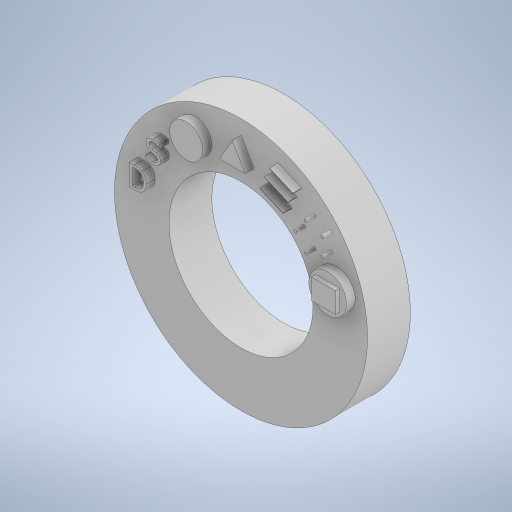
# Autodesk Inventor part: lab5CADfiguras
Saved by Autodesk Inventor 2023 (Build 270158000, 158)
## iProperties
Created: 2022-10-28
Part Number: lab5CADfiguras
Material: Generic
Document SubType Name: Modeling
Designer: jhair
Density: 1 g/cm^3
Appearance: Default
Author: jhair
Autodesk Inventor part; units mm, degrees
ref_plane "YZ Plane" through (0, 0, 0) normal (1, 0, 0) x (0, 1, 0)
ref_plane "XZ Plane" through (0, 0, 0) normal (0, 1, 0) x (-1, 0, 0)
ref_plane "XY Plane" through (0, 0, 0) normal (0, 0, 1) x (1, 0, 0)
sketch "Sketch1" plane through (0, 0, 0) normal (0, 0, 1) x (1, 0, 0)
  circle A0 centre (0, 0) radius 295
  circle A1 centre (0, 0) radius 168
  dimension "d0" = 590
  dimension "d1" = 336
  constraints: 2 centre point, 2 coincident
  measures "d0" diameter of A0
  measures "d1" diameter of A1
extrude "Extrusion1" add sketch "Sketch1" along normal blind 100
sketch "Sketch2" plane through (0, 0, 100) normal (0, 0, 1) x (1, 0, 0)
  line L0 (-204.3933, 171.1712) -> (-160.5291, 171.1712) construction
  line L1 (-160.5291, 171.1712) -> (-160.5291, 111.0696) construction
  line L2 (-160.5291, 111.0696) -> (-204.3933, 111.0696) construction
  line L3 (-204.3933, 111.0696) -> (-204.3933, 171.1712) construction
  line L4 (-245.1262, 97.2034) -> (-201.262, 97.2034) construction
  line L5 (-201.262, 97.2034) -> (-201.262, 37.1018) construction
  line L6 (-201.262, 37.1018) -> (-245.1262, 37.1018) construction
  line L7 (-245.1262, 37.1018) -> (-245.1262, 97.2034) construction
  spline S0 degree 2 poles (-185.39, 119.3884) (-190.8195, 119.3884) (-198.437, 121.6574) (-201.8001, 123.2782) knots 0 0 0 1 2 2 2
  line L8 (-201.8001, 123.2782) -> (-201.8001, 131.625)
  line L9 (-201.8001, 131.625) -> (-201.3139, 131.625)
  spline S1 degree 2 poles (-201.3139, 131.625) (-198.0319, 128.5456) (-189.7255, 125.142) (-185.8763, 125.142) knots 0 0 0 1 2 2 2
  spline S2 degree 2 poles (-185.8763, 125.142) (-180.3657, 125.142) (-174.7336, 129.7206) (-174.7336, 133.4889) knots 0 0 0 1 2 2 2
  spline S3 degree 2 poles (-174.7336, 133.4889) (-174.7336, 136.4873) (-177.6915, 140.215) (-180.8925, 141.1469) knots 0 0 0 1 2 2 2
  spline S4 degree 2 poles (-180.8925, 141.1469) (-183.202, 141.7952) (-187.0513, 142.6866) (-189.9281, 143.4159) knots 0 0 0 1 2 2 2
  spline S5 degree 2 poles (-189.9281, 143.4159) (-192.5213, 144.1048) (-196.6137, 146.1712) (-198.1939, 147.8325) knots 0 0 0 1 2 2 2
  spline S6 degree 2 poles (-198.1939, 147.8325) (-199.7336, 149.4937) (-201.4354, 153.9508) (-201.4354, 156.8681) knots 0 0 0 1 2 2 2
  spline S7 degree 2 poles (-201.4354, 156.8681) (-201.4354, 162.9459) (-191.9541, 171.1712) (-184.6202, 171.1712) knots 0 0 0 1 2 2 2
  spline S8 degree 2 poles (-184.6202, 171.1712) (-180.4062, 171.1712) (-172.9508, 169.51) (-169.7498, 167.9297) knots 0 0 0 1 2 2 2
  line L10 (-169.7498, 167.9297) -> (-169.7498, 159.9881)
  line L11 (-169.7498, 159.9881) -> (-170.2361, 159.9881)
  spline S9 degree 2 poles (-170.2361, 159.9881) (-172.6267, 162.1761) (-180.0821, 165.4176) (-184.1745, 165.4176) knots 0 0 0 1 2 2 2
  spline S10 degree 2 poles (-184.1745, 165.4176) (-188.7936, 165.4176) (-194.5067, 161.0821) (-194.5067, 157.557) knots 0 0 0 1 2 2 2
  spline S11 degree 2 poles (-194.5067, 157.557) (-194.5067, 154.3965) (-191.1437, 150.6283) (-187.9832, 149.7774) knots 0 0 0 1 2 2 2
  spline S12 degree 2 poles (-187.9832, 149.7774) (-185.8763, 149.2101) (-179.758, 147.7514) (-177.732, 147.1437) knots 0 0 0 1 2 2 2
  spline S13 degree 2 poles (-177.732, 147.1437) (-172.5862, 145.5634) (-167.805, 139.202) (-167.805, 134.5424) knots 0 0 0 1 2 2 2
  spline S14 degree 2 poles (-167.805, 134.5424) (-167.805, 131.5845) (-170.1956, 125.9119) (-172.343, 123.9265) knots 0 0 0 1 2 2 2
  spline S15 degree 2 poles (-172.343, 123.9265) (-174.7336, 121.7385) (-180.8114, 119.3884) (-185.39, 119.3884) knots 0 0 0 1 2 2 2
  spline S16 degree 2 poles (-200.6367, 72.1629) (-200.6367, 65.3152) (-206.1877, 54.2942) (-210.8474, 51.2147) knots 0 0 0 1 2 2 2
  spline S17 degree 2 poles (-210.8474, 51.2147) (-214.6561, 48.8241) (-222.4762, 47.2034) (-228.554, 47.2034) knots 0 0 0 1 2 2 2
  line L12 (-228.554, 47.2034) -> (-240.0613, 47.2034)
  line L13 (-240.0613, 47.2034) -> (-240.0613, 97.2034)
  line L14 (-240.0613, 97.2034) -> (-228.6756, 97.2034)
  spline S18 degree 2 poles (-228.6756, 97.2034) (-221.6253, 97.2034) (-213.6027, 95.0964) (-210.7663, 93.2326) knots 0 0 0 1 2 2 2
  spline S19 degree 2 poles (-210.7663, 93.2326) (-205.9446, 90.0316) (-200.6367, 79.4562) (-200.6367, 72.1629) knots 0 0 0 1 2 2 2
  spline S20 degree 2 poles (-207.5654, 72.2439) (-207.5654, 77.9976) (-211.3741, 86.1418) (-215.1424, 88.4514) knots 0 0 0 1 2 2 2
  spline S21 degree 2 poles (-215.1424, 88.4514) (-217.8166, 90.0316) (-223.8539, 91.4498) (-228.3514, 91.4498) knots 0 0 0 1 2 2 2
  line L15 (-228.3514, 91.4498) -> (-233.4163, 91.4498)
  line L16 (-233.4163, 91.4498) -> (-233.4163, 52.957)
  line L17 (-233.4163, 52.957) -> (-228.3514, 52.957)
  spline S22 degree 2 poles (-228.3514, 52.957) (-223.9349, 52.957) (-217.2493, 54.3752) (-214.5346, 56.2796) knots 0 0 0 1 2 2 2
  spline S23 degree 2 poles (-214.5346, 56.2796) (-211.05, 58.6297) (-207.5654, 66.4092) (-207.5654, 72.2439) knots 0 0 0 1 2 2 2
  point P0 (0, 0)
  constraints: 4 other
extrude "Extrusion2" add sketch "Sketch2" along normal blind 20
sketch "Sketch3" plane through (0, 0, 100) normal (0, 0, 1) x (1, 0, 0)
  circle A0 centre (-107.4544, 206.725) radius 38.7006
  line L0 (0, 260.9541) -> (30, 208.9926)
  line L1 (0, 260.9541) -> (60, 260.9541) construction
  line L2 (30, 208.9926) -> (-30, 208.9926)
  line L3 (-30, 208.9926) -> (0, 260.9541)
  line L4 (74.2712, 223.542) -> (129.0294, 200.0839)
  line L5 (129.0294, 200.0839) -> (129.6987, 201.6462)
  line L6 (129.6987, 201.6462) -> (74.9405, 225.1043)
  line L7 (74.9405, 225.1043) -> (74.2712, 223.542)
  line L8 (74.2712, 223.542) -> (129.6987, 201.6462) construction
  line L9 (129.0294, 200.0839) -> (74.9405, 225.1043) construction
  line L10 (63.2876, 195.758) -> (118.0458, 172.2999)
  line L11 (118.0458, 172.2999) -> (118.7151, 173.8622)
  line L12 (118.7151, 173.8622) -> (63.9569, 197.3203)
  line L13 (63.9569, 197.3203) -> (63.2876, 195.758)
  line L14 (63.2876, 195.758) -> (118.7151, 173.8622) construction
  line L15 (118.0458, 172.2999) -> (63.9569, 197.3203) construction
  line L16 (86.0027, 247.306) -> (140.7609, 223.848)
  line L17 (140.7609, 223.848) -> (141.4302, 225.4103)
  line L18 (141.4302, 225.4103) -> (86.672, 248.8684)
  line L19 (86.672, 248.8684) -> (86.0027, 247.306)
  circle A1 centre (181.5681, 150.8575) radius 34.8144
  circle A2 centre (146.7537, 150.8575) radius 3.4311
  circle A3 centre (170.8099, 117.747) radius 3.4311
  circle A4 centre (209.7335, 130.3941) radius 3.4311
  circle A5 centre (209.7335, 171.3209) radius 3.4311
  circle A6 centre (170.8099, 183.9679) radius 3.4311
  circle A7 centre (222.3863, 63.4959) radius 44.0014
  line L20 (189.9505, 93.2287) -> (254.8222, 93.2287)
  line L21 (254.8222, 93.2287) -> (254.8222, 33.763)
  line L22 (254.8222, 33.763) -> (189.9505, 33.763)
  line L23 (189.9505, 33.763) -> (189.9505, 93.2287)
  line L24 (189.9505, 93.2287) -> (254.8222, 33.763) construction
  line L25 (254.8222, 93.2287) -> (189.9505, 33.763) construction
  point P0 (0, 0)
  point P1 (101.985, 212.5941)
  point P2 (91.0013, 184.8101)
  point P3 (189.9505, 93.2287)
  point P4 (189.9505, 93.2287)
  point P5 (254.8222, 93.2287)
  point P6 (254.8222, 93.2287)
  point P7 (189.9505, 33.763)
  point P8 (189.9505, 33.763)
  dimension "d6" = 60
  dimension "d7" = 60
  dimension "d8" = 60
  dimension "d9" = 60
  dimension "d12" = 360
  constraints: 52 end point, 8 parallel, 6 centre point, 6 midpoint, 4 perpendicular, 3 horizontal, 1 equal length, 1 horizontal alignment, 16 other
  measures "d6" distance of L0.start L0.end
  measures "d7" angle of L0 L1
  measures "d8" distance of L0.end L2.end
  measures "d9" angle of L0 L2
extrude "Extrusion3" add sketch "Sketch3" along normal blind 20 contours A0 | L0 L2 L3 | L7 L6 L5 L4 | L13 L12 L11 L10 | L19 L18 L17 L16 | A5 A1 | A1 A5 | A4 A1 | A1 A4 | A6 A1 | A1 A6 | A3 A1 | A1 A3 | A2 A1 | A1 A2 | A7 L21 | L20 A7 | L21 L22 L23 L20 | A7 L22 | L23 A7
sketch "Sketch4" plane through (222.3863, 63.4959, 120) normal (0, 0, 1) x (1, 0, 0)
  line L0 (-27.8414, 23.9777) -> (27.8414, 23.9777)
  line L1 (27.8414, 23.9777) -> (27.8414, -23.9777)
  line L2 (27.8414, -23.9777) -> (-27.8414, -23.9777)
  line L3 (-27.8414, -23.9777) -> (-27.8414, 23.9777)
  line L4 (-27.8414, 23.9777) -> (27.8414, -23.9777) construction
  line L5 (27.8414, 23.9777) -> (-27.8414, -23.9777) construction
  point P0 (-222.3863, -63.4959)
  point P1 (0, 0)
  constraints: 12 end point, 2 midpoint, 2 parallel, 1 horizontal, 1 perpendicular
extrude "Extrusion4" add sketch "Sketch4" along normal blind 10
body "Solid1"
